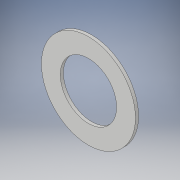
# Autodesk Inventor part: peca1
Saved by Autodesk Inventor 2019 (Build 230136000, 136)
## iProperties
Created: 2019-04-16
Part Number: peca1
Material: Generic
Document SubType Name: Modeling
Designer: Vladimir
Density: 1 g/cm^3
Appearance: Default
Author: Vladimir
Autodesk Inventor part; units mm, degrees
ref_plane "YZ Plane" through (0, 0, 0) normal (1, 0, 0) x (0, 1, 0)
ref_plane "XZ Plane" through (0, 0, 0) normal (0, 1, 0) x (-1, 0, 0)
ref_plane "XY Plane" through (0, 0, 0) normal (0, 0, 1) x (1, 0, 0)
sketch "Sketch1" plane through (0, 0, 0) normal (0, 0, 1) x (1, 0, 0)
  circle A0 centre (0, 0) radius 18
  circle A1 centre (0, 0) radius 30
  dimension "d0" = 36
  dimension "d4" = 60
  constraints: 2 centre point, 2 coincident
  measures "d0" diameter of A0
  measures "d4" diameter of A1
extrude "Extrusion1" add sketch "Sketch1" along normal blind 2
body "Solid1"
